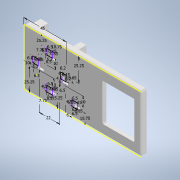
# Autodesk Inventor part: Upper_Half
Saved by Autodesk Inventor 2022 (Build 260153000, 153)
## iProperties
Created: 2023-09-02
Part Number: Upper_Half
Material: Generic
Document SubType Name: Modeling
Designer: Petr Černý
Density: 1 g/cm^3
Appearance: Default
Author: Petr Černý
Autodesk Inventor part; units mm, degrees
ref_plane "YZ Plane" through (0, 0, 0) normal (1, 0, 0) x (0, 1, 0)
ref_plane "XZ Plane" through (0, 0, 0) normal (0, 1, 0) x (-1, 0, 0)
ref_plane "XY Plane" through (0, 0, 0) normal (0, 0, 1) x (1, 0, 0)
sketch "Sketch1" plane through (0, 0, 0) normal (0, 0, 1) x (1, 0, 0)
  line L0 (110.9399, 39.6241) -> (-14.0601, 39.6241)
  line L1 (-14.0601, 39.6241) -> (-14.0601, -20.3759)
  line L2 (-14.0601, -20.3759) -> (110.9399, -20.3759)
  line L3 (110.9399, -20.3759) -> (110.9399, 39.6241)
  point P0 (0, 0)
  dimension "d0" = 125
  dimension "d1" = 60
  constraints: 8 end point, 2 parallel, 1 horizontal, 1 perpendicular
  measures "d0" distance of L1.end L2.end
  measures "d1" distance of L0.end L1.end
extrude "Extrusion1" add sketch "Sketch1" along normal blind 6
shell "Shell1" thickness 2 removed faces 1 at (27.6065, 19.6241, 0)
sketch "Sketch4" plane through (0, 0, 6) normal (0, 0, 1) x (1, 0, 0)
  line L0 (-14.0601, 39.6241) -> (-14.0601, -20.3759) projected
  line L1 (110.9399, 39.6241) -> (-14.0601, 39.6241) projected
  line L2 (-14.0601, -20.3759) -> (110.9399, -20.3759) projected
  line L3 (30.7899, 15.2241) -> (24.5899, 15.2241)
  line L4 (24.5899, 15.2241) -> (24.5899, 9.0241)
  line L5 (24.5899, 9.0241) -> (30.7899, 9.0241)
  line L6 (30.7899, 9.0241) -> (30.7899, 15.2241)
  line L7 (43.225, -4.2759) -> (37.025, -4.2759)
  line L8 (37.025, -4.2759) -> (37.025, -10.4759)
  line L9 (37.025, -10.4759) -> (43.225, -10.4759)
  line L10 (43.225, -10.4759) -> (43.225, -4.2759)
  line L11 (16.5351, -4.2759) -> (10.3351, -4.2759)
  line L12 (10.3351, -4.2759) -> (10.3351, -10.4759)
  line L13 (10.3351, -10.4759) -> (16.5351, -10.4759)
  line L14 (16.5351, -10.4759) -> (16.5351, -4.2759)
  line L15 (16.5378, 29.7241) -> (10.3378, 29.7241)
  line L16 (10.3378, 29.7241) -> (10.3378, 23.5241)
  line L17 (10.3378, 23.5241) -> (16.5378, 23.5241)
  line L18 (16.5378, 23.5241) -> (16.5378, 29.7241)
  line L19 (1.3347, 15.2241) -> (-4.8653, 15.2241)
  line L20 (-4.8653, 15.2241) -> (-4.8653, 9.0241)
  line L21 (-4.8653, 9.0241) -> (1.3347, 9.0241)
  line L22 (1.3347, 9.0241) -> (1.3347, 15.2241)
  point P0 (0, 0)
  point P1 (-1.8219, 8.778)
  point P2 (-4.0601, 4.8741)
  point P3 (2.4073, 5.5241)
  point P4 (1.4847, 14.3741)
  point P5 (10.2177, -4.4759)
  point P6 (10.1573, -8.9755)
  point P7 (16.6573, -8.9755)
  point P8 (16.6851, -5.1259)
  point P9 (16.6878, 28.8741)
  point P10 (15.7347, 24.3741)
  point P11 (9.2347, 24.3741)
  point P12 (10.1886, 28.7718)
  point P13 (30.9399, 14.3741)
  point P14 (27.1034, 9.127)
  point P15 (24.4073, 5.5241)
  point P16 (30.875, 4.8771)
  point P17 (43.4398, -9.6259)
  point P18 (36.9398, -9.6224)
  point P19 (36.875, -5.1229)
  point P20 (43.375, -5.1229)
  dimension "d30" = 4.5
  dimension "d31" = 6.5
  dimension "d32" = 6.5
  dimension "d33" = 10
  dimension "d34" = 25.25
  dimension "d35" = 4.5
  dimension "d36" = 6.5
  dimension "d37" = 6.5
  dimension "d38" = 4.5
  dimension "d39" = 6.5
  dimension "d40" = 6.5
  dimension "d41" = 4.5
  dimension "d42" = 6.5
  dimension "d43" = 6.5
  dimension "d44" = 22
  dimension "d45" = 0
  dimension "d46" = 7.75
  dimension "d47" = 7.75
  dimension "d48" = 10
  dimension "d49" = 10
  dimension "d71" = 4.5
  dimension "d72" = 6.5
  dimension "d73" = 6.5
  dimension "d74" = 10
  dimension "d75" = 6
  dimension "d81" = 6.2
  dimension "d82" = 6.2
  dimension "d85" = 45
  dimension "d86" = 0.15
  dimension "d87" = 25.25
  dimension "d88" = 0.85
  dimension "d89" = 6.2
  dimension "d90" = 6.2
  dimension "d91" = 6.2
  dimension "d92" = 6.2
  dimension "d93" = 6.2
  dimension "d94" = 6.2
  dimension "d95" = 10.75
  dimension "d96" = 0.85
  dimension "d98" = 0.15
  dimension "d99" = 6.2
  dimension "d100" = 6.2
  dimension "d101" = 15.25
  dimension "d102" = 0.15
  dimension "d103" = 0.85
  dimension "d104" = 10.75
  dimension "d105" = 0.15
  dimension "d106" = 0.85
  dimension "d107" = 25.25
  dimension "d108" = 0.15
  dimension "d109" = 0.85
  constraints: 40 end point, 10 parallel, 5 horizontal, 5 perpendicular
  measures "d30" distance of point (-4.06, 4.874) point (-1.822, 8.778)
  measures "d31" distance of point (1.485, 14.374) point (-1.822, 8.778)
  measures "d32" distance of point (2.407, 5.524) point (-4.06, 4.874)
  measures "d33" distance from line of L0 point (-4.06, 4.874)
  measures "d34" distance from line of L2 point (-4.06, 4.874)
  measures "d35" distance of point (10.157, -8.975) point (10.218, -4.476)
  measures "d36" distance of point (16.685, -5.126) point (10.218, -4.476)
  measures "d37" distance of point (16.657, -8.975) point (10.157, -8.975)
  measures "d38" distance of point (9.235, 24.374) point (10.189, 28.772)
  measures "d39" distance of point (16.688, 28.874) point (10.189, 28.772)
  measures "d40" distance of point (15.735, 24.374) point (9.235, 24.374)
  measures "d41" distance of point (24.407, 5.524) point (27.103, 9.127)
  measures "d42" distance of point (30.94, 14.374) point (27.103, 9.127)
  measures "d43" distance of point (30.875, 4.877) point (24.407, 5.524)
  measures "d44" distance of point (24.407, 5.524) point (2.407, 5.524)
  measures "d45" vertical distance of point (24.407, 5.524) point (2.407, 5.524)
  measures "d46" horizontal distance of point (10.157, -8.975) point (2.407, 5.524)
  measures "d47" horizontal distance of point (9.235, 24.374) point (1.485, 14.374)
  measures "d48" vertical distance of point (1.485, 14.374) point (9.235, 24.374)
  measures "d49" vertical distance of point (10.218, -4.476) point (2.407, 5.524)
  measures "d71" distance of point (36.94, -9.622) point (36.875, -5.123)
  measures "d72" distance of point (43.375, -5.123) point (36.875, -5.123)
  measures "d73" distance of point (43.44, -9.626) point (36.94, -9.622)
  measures "d74" vertical distance of point (36.875, -5.123) point (30.875, 4.877)
  measures "d75" horizontal distance of point (30.875, 4.877) point (36.875, -5.123)
  measures "d81" distance between parallel lines of L4 L6
  measures "d82" distance of L5.end L3.start
  measures "d85" distance from line of L0 point (30.94, 14.374)
  measures "d86" distance from line of point (30.94, 14.374) L6
  measures "d87" distance from line of L1 point (30.94, 14.374)
  measures "d88" distance from line of point (30.94, 14.374) L3
  measures "d89" distance of L9.end L8.end
  measures "d90" distance of L8.end L7.end
  measures "d91" distance of L17.end L16.end
  measures "d92" distance of L16.end L15.end
  measures "d93" distance of L21.end L20.end
  measures "d94" distance of L20.end L19.end
  measures "d95" distance from line of L2 point (43.44, -9.626)
  measures "d96" distance from line of L9 point (43.44, -9.626)
  measures "d98" distance from line of L10 point (43.375, -5.123)
  measures "d99" distance of L12.end L13.end
  measures "d100" distance of L11.end L12.end
  measures "d101" distance from line of L2 point (16.685, -5.126)
  measures "d102" distance from line of L14 point (16.685, -5.126)
  measures "d103" distance from line of point (16.685, -5.126) L11
  measures "d104" distance from line of L1 point (16.688, 28.874)
  measures "d105" distance from line of L18 point (16.688, 28.874)
  measures "d106" distance from line of point (16.688, 28.874) L15
  measures "d107" distance from line of point (1.485, 14.374) L1
  measures "d108" distance from line of point (1.485, 14.374) L22
  measures "d109" distance from line of point (1.485, 14.374) L19
sketch "Sketch5" plane through (108.9399, -18.3759, 4) normal (0, 0, -1) x (-1, 0, 0)
  line L0 (0, 0) -> (0, 56) projected
  line L1 (0, 0) -> (46.7, 0)
  line L2 (0, 51) -> (0, 0)
  line L3 (0, 0) -> (0, 56) projected
  line L4 (0, 2.5) -> (46.7, 2.5)
  line L5 (46.7, 2.5) -> (46.7, 53.5)
  line L6 (46.7, 53.5) -> (0, 53.5)
  line L7 (0, 53.5) -> (0, 2.5)
  line L8 (0, 56) -> (121, 56) projected
  point P0 (108.9399, 18.3759)
  point P1 (0, 53.5)
  dimension "d124" = 46.7
  dimension "d125" = 51
  dimension "d126" = 2.5
  constraints: 12 end point, 2 horizontal, 2 parallel, 1 perpendicular, 1 point on line
  measures "d124" distance of L6.end L5.end
  measures "d125" distance of L5.end L4.end
  measures "d126" distance between parallel lines of L6 L8
extrude "Extrusion3" add sketch "Sketch5" along normal blind 2
sketch "Sketch6" plane through (108.9399, -18.3759, 2) normal (0, 0, -1) x (-1, 0, 0)
  line L0 (5.2, 8.05) -> (39.2, 8.05)
  line L1 (39.2, 8.05) -> (39.2, 47.95)
  line L2 (39.2, 47.95) -> (5.2, 47.95)
  line L3 (5.2, 47.95) -> (5.2, 8.05)
  line L4 (0, 0) -> (0, 56) projected
  line L5 (121, 0) -> (0, 0) projected
  line L6 (0, 56) -> (121, 56) projected
  point P0 (108.9399, 18.3759)
  point P1 (72, 0)
  point P2 (72, 56)
  dimension "d60" = 34
  dimension "d61" = 39.9
  dimension "d62" = 8.05
  dimension "d63" = 5.2
  constraints: 8 end point, 2 parallel, 1 horizontal, 1 perpendicular
  measures "d60" distance of L2.end L1.end
  measures "d61" distance of L1.end L0.end
  measures "d62" distance between parallel lines of L5 L0
  measures "d63" distance between parallel lines of L3 L4
extrude "Extrusion4" cut sketch "Sketch6" against normal through all
fillet "Fillet1" radius 2 8 edges at (-14.0601, 9.6241, 6) (48.4399, -20.3759, 6) (110.9399, 9.6241, 6) (48.4399, 39.6241, 6) (-14.0601, -20.3759, 3) (-14.0601, 39.6241, 3) (110.9399, -20.3759, 3) (110.9399, 39.6241, 3)
fillet "Fillet2" radius 1 4 edges at (103.7399, 29.5741, 4) (69.7399, 29.5741, 4) (69.7399, -10.3259, 4) (103.7399, -10.3259, 4)
fillet "Fillet7" radius 2 2 edges at (108.9399, 37.6241, 2) (108.9399, -18.3759, 2)
sketch "Sketch11" plane through (-12.0601, -18.3759, 4) normal (0, 0, -1) x (-1, 0, 0)
  line L0 (0, 56) -> (-121, 56) projected
  line L1 (0, 56) -> (-8, 56)
  line L2 (-8, 56) -> (-8, 48)
  line L3 (-8, 48) -> (0, 48)
  line L4 (0, 48) -> (0, 56)
  line L5 (-42.5, 56) -> (-48.5, 56)
  line L6 (-48.5, 56) -> (-48.5, 48)
  line L7 (-48.5, 48) -> (-42.5, 48)
  line L8 (-42.5, 48) -> (-42.5, 56)
  line L9 (0, 0) -> (-119, 0) projected
  line L10 (-48.5, 0) -> (-42.5, 0)
  line L11 (-42.5, 0) -> (-42.5, 13)
  line L12 (-42.5, 13) -> (-48.5, 13)
  line L13 (-48.5, 13) -> (-48.5, 0)
  line L14 (0, 0) -> (-8, 0)
  line L15 (-8, 0) -> (-8, 12)
  line L16 (-8, 12) -> (0, 12)
  line L17 (0, 12) -> (0, 0)
  point P0 (-12.0601, 18.3759)
  point P1 (-42.5, 0)
  dimension "d127" = 8
  dimension "d128" = 8
  dimension "d129" = 6
  dimension "d130" = 8
  dimension "d131" = 6
  dimension "d132" = 13
  dimension "d133" = 8
  dimension "d134" = 12
  dimension "d135" = 34.5
  dimension "d136" = 34.5
  constraints: 32 end point, 8 parallel, 4 horizontal, 4 perpendicular, 2 point on line
  measures "d127" distance of L3.end L2.end
  measures "d128" distance of L2.end L1.end
  measures "d129" distance of L7.end L6.end
  measures "d130" distance of L6.end L5.end
  measures "d131" distance of L12.end L11.end
  measures "d132" distance of L11.end L10.end
  measures "d133" distance of L15.end L16.end
  measures "d134" distance of L14.end L15.end
  measures "d135" distance between parallel lines of L8 L2
  measures "d136" distance between parallel lines of L11 L15
extrude "Extrusion7" add sketch "Sketch11" along normal blind 14
sketch "Sketch12" plane through (-12.0601, -18.3759, -10) normal (0, 0, -1) x (-1, 0, 0)
  circle A0 centre (-5, 51.5) radius 1.5 projected
  circle A1 centre (-5, 9.4) radius 1.5 projected
  circle A2 centre (-45, 9.4) radius 1.5 projected
  circle A3 centre (-45, 51.55) radius 1.6 projected
  point P0 (-12.0601, 18.3759)
  constraints: 4 coincident
hole "Hole4" at (32.9399, 33.1741, -10) at (32.9399, -8.9759, -10) at (-7.0601, -8.9759, -10) at (-7.0601, 33.1241, -10) direction (0, 0, 1) diameter 2.459 depth 8.8 tip angle 118 thread size "M3x0.5" class "6H" standard "ISO Metric profile"
sketch "Sketch13" plane through (0, 0, 6) normal (0, 0, 1) x (1, 0, 0)
  line L0 (6.9399, 12.6241) -> (0.9399, 12.6241)
  line L1 (0.9399, 12.6241) -> (0.9399, 6.6241)
  line L2 (0.9399, 6.6241) -> (6.9399, 6.6241)
  line L3 (6.9399, 6.6241) -> (6.9399, 12.6241)
  line L4 (108.9399, 39.6241) -> (-12.0601, 39.6241) projected
  line L5 (-14.0601, 37.6241) -> (-14.0601, -18.3759) projected
  line L6 (32.9399, 12.6241) -> (26.9399, 12.6241)
  line L7 (26.9399, 12.6241) -> (26.9399, 6.6241)
  line L8 (26.9399, 6.6241) -> (32.9399, 6.6241)
  line L9 (32.9399, 6.6241) -> (32.9399, 12.6241)
  line L10 (-12.0601, -20.3759) -> (108.9399, -20.3759) projected
  line L11 (19.9399, 28.6241) -> (13.9399, 28.6241)
  line L12 (13.9399, 28.6241) -> (13.9399, 22.6241)
  line L13 (13.9399, 22.6241) -> (19.9399, 22.6241)
  line L14 (19.9399, 22.6241) -> (19.9399, 28.6241)
  line L15 (19.9399, -3.3759) -> (13.9399, -3.3759)
  line L16 (13.9399, -3.3759) -> (13.9399, -9.3759)
  line L17 (13.9399, -9.3759) -> (19.9399, -9.3759)
  line L18 (19.9399, -9.3759) -> (19.9399, -3.3759)
  line L19 (45.9399, -3.3759) -> (39.9399, -3.3759)
  line L20 (39.9399, -3.3759) -> (39.9399, -9.3759)
  line L21 (39.9399, -9.3759) -> (45.9399, -9.3759)
  line L22 (45.9399, -9.3759) -> (45.9399, -3.3759)
  point P0 (0, 0)
  dimension "d146" = 6
  dimension "d147" = 6
  dimension "d148" = 27
  dimension "d149" = 15
  dimension "d150" = 6
  dimension "d151" = 6
  dimension "d152" = 20
  dimension "d153" = 27
  dimension "d154" = 6
  dimension "d155" = 6
  dimension "d156" = 7
  dimension "d157" = 10
  dimension "d158" = 6
  dimension "d159" = 6
  dimension "d160" = 10
  dimension "d161" = 7
  dimension "d162" = 6
  dimension "d163" = 6
  dimension "d164" = 7
  dimension "d165" = 10
  constraints: 40 end point, 10 parallel, 5 horizontal, 5 perpendicular
  measures "d146" distance of L2.end L1.end
  measures "d147" distance of L1.end L0.end
  measures "d148" distance between parallel lines of L0 L4
  measures "d149" distance between parallel lines of L5 L1
  measures "d150" distance of L8.end L7.end
  measures "d151" distance of L7.end L6.end
  measures "d152" distance between parallel lines of L7 L3
  measures "d153" distance between parallel lines of L10 L8
  measures "d154" distance of L13.end L12.end
  measures "d155" distance of L12.end L11.end
  measures "d156" distance between parallel lines of L12 L3
  measures "d157" distance between parallel lines of L0 L13
  measures "d158" distance of L17.end L16.end
  measures "d159" distance of L16.end L15.end
  measures "d160" distance between parallel lines of L15 L2
  measures "d161" distance between parallel lines of L3 L16
  measures "d162" distance of L21.end L19.start
  measures "d163" distance of L20.end L21.end
  measures "d164" distance between parallel lines of L20 L9
  measures "d165" distance between parallel lines of L19 L8
extrude "Extrusion8" cut sketch "Sketch13" against normal blind 3
sketch "Sketch14" plane through (108.9399, 35.1241, 4) normal (0, 0, -1) x (-1, 0, 0)
  line L0 (2, 2.5) -> (72.5, 2.5) projected
  circle A0 centre (76, -1.95) radius 1.2295 projected
  line L1 (78.5, -5.5) -> (78.5, 2.5) projected
  line L2 (78.5, 2.5) -> (72.5, 2.5) projected
  line L3 (72.5, 2.5) -> (72.5, -5.5) projected
  line L4 (72.5, -5.5) -> (78.5, -5.5) projected
  circle A1 centre (116, -2) radius 1.2295 projected
  line L5 (121, 2.5) -> (113, 2.5) projected
  line L6 (113, 2.5) -> (113, -5.5) projected
  line L7 (113, -5.5) -> (121, -5.5) projected
  line L8 (121, -5.5) -> (121, 2.5) projected
  line L9 (78.5, 2.5) -> (113, 2.5) projected
  line L10 (121, -5.5) -> (121, -41.5) projected
  circle A2 centre (116, -44.1) radius 1.2295 projected
  line L11 (121, -41.5) -> (113, -41.5) projected
  line L12 (113, -41.5) -> (113, -53.5) projected
  line L13 (113, -53.5) -> (121, -53.5) projected
  line L14 (121, -53.5) -> (121, -41.5) projected
  line L15 (113, -53.5) -> (78.5, -53.5) projected
  circle A3 centre (76, -44.1) radius 1.2295 projected
  line L16 (72.5, -40.5) -> (72.5, -53.5) projected
  line L17 (72.5, -53.5) -> (78.5, -53.5) projected
  line L18 (78.5, -53.5) -> (78.5, -40.5) projected
  line L19 (78.5, -40.5) -> (72.5, -40.5) projected
  line L20 (72.5, -53.5) -> (2, -53.5) projected
  line L21 (0, -51) -> (46.7, -51) projected
  line L22 (46.7, -51) -> (46.7, 0) projected
  line L23 (46.7, 0) -> (0, 0) projected
  line L24 (6.2, -5.55) -> (38.2, -5.55) projected
  arc A4 (39.2, -6.55) -> (38.2, -5.55) centre (38.2, -6.55) ccw projected
  line L25 (39.2, -6.55) -> (39.2, -44.45) projected
  arc A5 (38.2, -45.45) -> (39.2, -44.45) centre (38.2, -44.45) ccw projected
  line L26 (38.2, -45.45) -> (6.2, -45.45) projected
  arc A6 (5.2, -44.45) -> (6.2, -45.45) centre (6.2, -44.45) ccw projected
  line L27 (5.2, -44.45) -> (5.2, -6.55) projected
  arc A7 (6.2, -5.55) -> (5.2, -6.55) centre (6.2, -6.55) ccw projected
  line L28 (0, 0) -> (46.7, 0) projected
  arc A8 (2, 2.5) -> (0, 0.5) centre (2, 0.5) ccw projected
  line L29 (0, 0) -> (0, 0.5)
  arc A9 (2, 2.5) -> (0, 0.5) centre (2, 0.5) ccw
  line L30 (2, 2.5) -> (72.5, 2.5) projected
  line L31 (2, 2.5) -> (72.5, 2.5)
  line L32 (72.5, -5.5) -> (72.5, 2.5) projected
  line L33 (72.5, 2.5) -> (72.5, -5.5)
  line L34 (78.5, -5.5) -> (72.5, -5.5) projected
  line L35 (72.5, -5.5) -> (78.5, -5.5)
  line L36 (78.5, 2.5) -> (78.5, -5.5) projected
  line L37 (78.5, -5.5) -> (78.5, 2.5)
  line L38 (78.5, 2.5) -> (113, 2.5)
  line L39 (113, -5.5) -> (113, 2.5) projected
  line L40 (121, -5.5) -> (113, -5.5) projected
  line L41 (113, -5.5) -> (121, -5.5)
  line L42 (113, -41.5) -> (121, -41.5) projected
  line L43 (121, -5.5) -> (121, -41.5)
  line L44 (121, -41.5) -> (113, -41.5)
  line L45 (113, -53.5) -> (113, -41.5) projected
  line L46 (113, -53.5) -> (78.5, -53.5)
  line L47 (78.5, -40.5) -> (78.5, -53.5) projected
  line L48 (72.5, -40.5) -> (78.5, -40.5) projected
  line L49 (78.5, -40.5) -> (72.5, -40.5)
  line L50 (72.5, -53.5) -> (72.5, -40.5) projected
  line L51 (72.5, -40.5) -> (72.5, -53.5)
  arc A10 (0, -51.5) -> (2, -53.5) centre (2, -51.5) ccw projected
  line L52 (72.5, -53.5) -> (2, -53.5)
  arc A11 (0, -51) -> (2, -53.5) centre (2, -51.45) ccw
  line L53 (46.7, -51) -> (0, -51) projected
  line L54 (0, -51) -> (46.7, -51)
  line L55 (46.7, 0) -> (46.7, -51) projected
  line L56 (46.7, -51) -> (46.7, 0)
  line L57 (0, 0) -> (0, 0.5) projected
  line L58 (46.7, 0) -> (0, 0)
  line L59 (0, -51) -> (0, 0) projected
  point P0 (108.9399, -35.1241)
  point P1 (1, 0)
  point P2 (1, -51)
  point P3 (78.5, -53.5)
  point P4 (72.5, 2.5)
  point P5 (0, -51)
  constraints: 32 end point, 12 perpendicular, 5 tangent, 4 point on circle, 2 centre point, 2 horizontal, 1 collinear, 1 point on line, 1 vertical
extrude "Extrusion9" add sketch "Sketch14" along normal blind 2 contours L0 L3 L4 L1 L9 L6 L7 L10 L11 L12 L15 L18 L19 L16 L20 A11 L21 L22 L23 L29 A8
body "Solid1"
